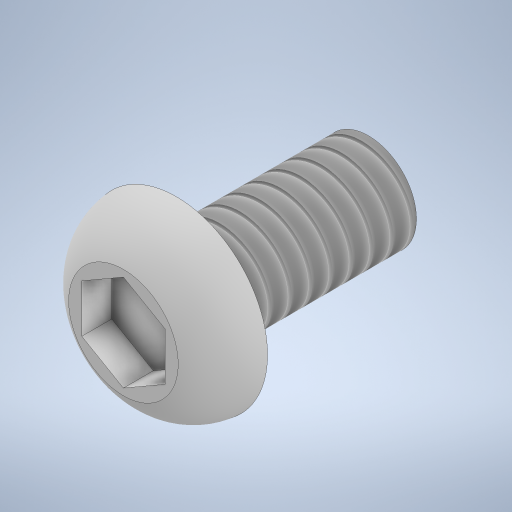
# Autodesk Inventor part: 5mm Button Head Screw Botch
Saved by Autodesk Inventor 2023.5 (Build 275446000, 446)
## iProperties
Created: 2024-08-12
Part Number: 5mm Button Head Screw Botch
Material: Generic
Document SubType Name: Modeling
Designer: punny
Density: 1 g/cm^3
Appearance: Default
Author: punny
Autodesk Inventor part; units mm, degrees
ref_plane "YZ Plane" through (0, 0, 0) normal (1, 0, 0) x (0, 1, 0)
ref_plane "XZ Plane" through (0, 0, 0) normal (0, 1, 0) x (-1, 0, 0)
ref_plane "XY Plane" through (0, 0, 0) normal (0, 0, 1) x (1, 0, 0)
sketch "Sketch1" plane through (0, 0, 0) normal (0, 0, 1) x (1, 0, 0)
  circle A0 centre (0, 0) radius 2.5
  dimension "d0" = 5
  constraints: 1 centre point, 1 coincident
  measures "d0" diameter of A0
extrude "Extrusion1" add sketch "Sketch1" along normal blind 10
thread "Thread1" size "12-24 UNC" class "2A" standard "ANSI Unified Screw Threads" full length
sketch "Sketch2" plane through (0, 0, 0) normal (0, 1, 0) x (-1, 0, 0)
  line L0 (0, 10.0728) -> (-4.75, 10.0728)
  line L1 (2.5, 10) -> (-2.5, 10) projected
  line L2 (0, 10) -> (-4.75, 10)
  line L3 (0, 10) -> (0, 12.75)
  line L4 (0, 12.75) -> (-2.85, 12.75)
  arc A0 (-2.85, 12.75) -> (-4.75, 10) centre (-1.457, 9.7562) ccw
  point P0 (0, 0)
  dimension "d5" = 4.75
  dimension "d6" = 2.75
  dimension "d7" = 2.85
  dimension "d8" = 3.302
  constraints: 8 end point, 2 horizontal, 2 perpendicular, 2 point on circle, 1 centre point, 1 midpoint
  measures "d5" distance of L0.start L0.end
  measures "d6" distance of L2.start L3.end
  measures "d7" distance of L3.end L4.end
  measures "d8" radius of A0
revolve "Revolution1" add sketch "Sketch2" angle 360 about axis through (0, 0, 10) along (0, 0, 1)
sketch "Sketch3" plane through (0, 0, 12.75) normal (0, 0, 1) x (1, 0, 0)
  circle A0 centre (0, 0) radius 2.5 projected
  line L0 (0, 2.5) -> (2.1651, 1.25)
  line L1 (2.1651, 1.25) -> (2.1651, -1.25)
  line L2 (2.1651, -1.25) -> (0, -2.5)
  line L3 (0, -2.5) -> (-2.1651, -1.25)
  line L4 (-2.1651, -1.25) -> (-2.1651, 1.25)
  line L5 (-2.1651, 1.25) -> (0, 2.5)
  constraints: 12 end point, 1 coincident, 1 vertical alignment, 14 other
extrude "Extrusion2" cut sketch "Sketch3" against normal blind 1.56 contours L1 L2 L3 L4 L5 L0
body "Solid1"
